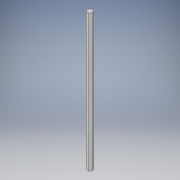
# Autodesk Inventor part: HexShaft12in
Saved by Autodesk Inventor 2018 (Build 220112000, 112)
## iProperties
Created: 2019-02-27
Part Number: HexShaft12in
Material: Generic
Document SubType Name: Modeling
Designer: snipe
Density: 1 g/cm^3
Appearance: Default
Author: snipe
Autodesk Inventor part; units mm, degrees
ref_plane "YZ Plane" through (0, 0, 0) normal (1, 0, 0) x (0, 1, 0)
ref_plane "XZ Plane" through (0, 0, 0) normal (0, 1, 0) x (-1, 0, 0)
ref_plane "XY Plane" through (0, 0, 0) normal (0, 0, 1) x (1, 0, 0)
sketch "Sketch1" plane through (0, 0, 0) normal (0, 1, 0) x (-1, 0, 0)
  line L0 (0, -7.699) -> (0, 7.699) projected
  line L1 (-8.89, 0) -> (8.89, 0) projected
  line L2 (8.89, 0) -> (-8.89, 0) projected
  line L3 (0, -7.699) -> (0, 7.699) projected
  line L4 (-6.35, 0) -> (-3.175, 5.4993)
  line L5 (-3.175, 5.4993) -> (3.175, 5.4993)
  line L6 (3.175, 5.4993) -> (6.35, 0)
  line L7 (6.35, 0) -> (3.175, -5.4993)
  line L8 (3.175, -5.4993) -> (-3.175, -5.4993)
  line L9 (-3.175, -5.4993) -> (-6.35, 0)
  point P0 (0, 0)
  point P1 (0, 0)
  dimension "d0" = 12.7
  constraints: 12 end point, 1 coincident, 1 point on line, 13 other
  measures "d0" distance of L4.start L6.end
extrude "Extrusion1" add sketch "Sketch1" along normal blind 304.8
body "Solid1"
